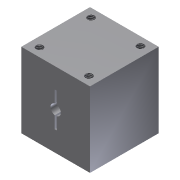
# Autodesk Inventor part: JointD1
Saved by Autodesk Inventor 2011 SP1 (Build 150282100, 282)
## iProperties
Created: 2012-10-24
Part Number: JointD1
Document SubType Name: Modeling
Designer: arihon
Density: 1 g/cm^3
Author: arihon
Autodesk Inventor part; units mm, degrees
ref_plane "YZ Plane" through (0, 0, 0) normal (1, 0, 0) x (0, 1, 0)
ref_plane "XZ Plane" through (0, 0, 0) normal (0, 1, 0) x (-1, 0, 0)
ref_plane "XY Plane" through (0, 0, 0) normal (0, 0, 1) x (1, 0, 0)
sketch "スケッチ1" plane through (0, 0, 0) normal (0, 0, 1) x (1, 0, 0)
  line L0 (-10, 10) -> (10, 10)
  line L1 (10, 10) -> (10, -10)
  line L2 (10, -10) -> (-10, -10)
  line L3 (-10, -10) -> (-10, 10)
  point P0 (0, 0)
  dimension "d0" = 20
  dimension "d1" = 10
  dimension "d2" = 20
  dimension "d3" = 10
  constraints: 8 end point, 2 parallel, 1 horizontal, 1 perpendicular
  measures "d0" distance of L0.start L0.end
  measures "d1" distance from line of L3 point (0, 0)
  measures "d2" distance of L2.end L0.start
  measures "d3" distance from line of L2 point (0, 0)
extrude "押し出し1" add sketch "スケッチ1" along normal blind 21.8
sketch "スケッチ2" plane through (0, 0, 21.8) normal (0, 0, 1) x (1, 0, 0)
  point P0 (0, 0)
  point P1 (-7.2, 7.5)
  point P2 (-7.2, -7.5)
  point P3 (7.2, -7.5)
  point P4 (7.2, 7.5)
  dimension "d6" = 14.4
  dimension "d7" = 14.4
  dimension "d8" = 15
  dimension "d9" = 15
  dimension "d10" = 7.2
  dimension "d11" = 7.2
  dimension "d12" = 7.5
  dimension "d13" = 7.5
  measures "d6" distance of point (7.2, 7.5) point (-7.2, 7.5)
  measures "d7" distance of point (-7.2, -7.5) point (7.2, -7.5)
  measures "d8" distance of point (-7.2, -7.5) point (-7.2, 7.5)
  measures "d9" distance of point (7.2, -7.5) point (7.2, 7.5)
  measures "d10" horizontal distance of point (-7.2, 7.5) point (0, 0)
  measures "d11" horizontal distance of point (-7.2, -7.5) point (0, 0)
  measures "d12" vertical distance of point (0, 0) point (-7.2, 7.5)
  measures "d13" vertical distance of point (0, 0) point (7.2, 7.5)
hole "Hole1" at (-7.2, 7.5, 21.8) at (-7.2, -7.5, 21.8) at (7.2, -7.5, 21.8) at (7.2, 7.5, 21.8) direction (0, 0, -1) diameter 2.013 end through all thread size "M2.5x0.45" class "6H" standard "ISO Metric profile"
sketch "スケッチ3" plane through (-10, -10, 0) normal (0, -1, 0) x (1, 0, 0)
  line L0 (20, 21.8) -> (0, 21.8) projected
  line L1 (20, 0) -> (20, 21.8) projected
  circle A0 centre (10, 10.9) radius 1.5
  line L2 (9.75, 15.9) -> (10.25, 15.9)
  line L3 (10.25, 15.9) -> (10.25, 5.9)
  line L4 (10.25, 5.9) -> (9.75, 5.9)
  line L5 (9.75, 5.9) -> (9.75, 15.9)
  point P0 (10, 0)
  dimension "d21" = 3
  dimension "d22" = 10.9
  dimension "d23" = 10
  dimension "d24" = 10
  dimension "d25" = 0.5
  dimension "d26" = 0.25
  dimension "d27" = 5
  constraints: 8 end point, 2 parallel, 1 centre point, 1 horizontal, 1 perpendicular
  measures "d21" diameter of A0
  measures "d22" distance from line of A0.centre L0
  measures "d23" distance from line of A0.centre L1
  measures "d24" distance of L4.end L2.start
  measures "d25" distance of L2.start L2.end
  measures "d26" distance from line of L5 A0.centre
  measures "d27" distance from line of L2 A0.centre
extrude "押し出し2" cut sketch "スケッチ3" against normal blind 15
equation "\"d1\" = 0.5 * d0"
equation "\"d3\" = 0.5 * d2"
equation "\"d7\" = d6"
equation "\"d9\" = d8"
equation "\"d10\" = 0.5 * d6"
equation "\"d11\" = d10"
equation "\"d12\" = 0.5 * d8"
equation "\"d13\" = d12"
equation "\"d26\" = 0.5 * d25"
equation "\"d27\" = 0.5 * d24"
